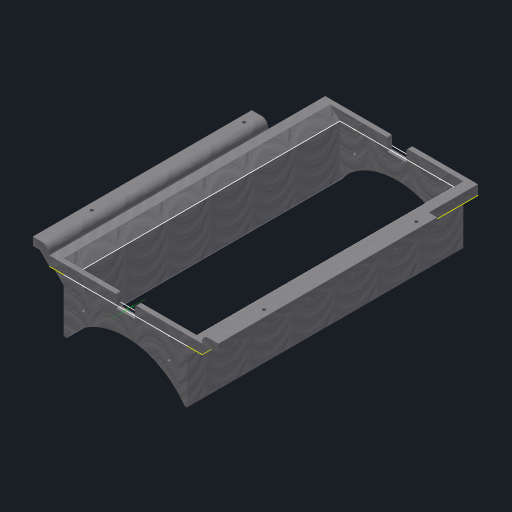
# Autodesk Inventor part: PUERTA_ACOPLE_ENTRADA_v2
Saved by Autodesk Inventor 2024.3 (Build 283343000, 343)
## iProperties
Created: 2024-07-11
Part Number: PUERTA_ACOPLE_ENTRADA_v2
Material: Steel, Mild, Welded
Document SubType Name: Modeling
Designer: Niler
Density: 7.85 g/cm^3
Appearance: Weld - Steel Mild
Author: Niler
Autodesk Inventor part; units mm, degrees
ref_plane "YZ Plane" through (0, 0, 0) normal (1, 0, 0) x (0, 1, 0)
ref_plane "XZ Plane" through (0, 0, 0) normal (0, 1, 0) x (-1, 0, 0)
ref_plane "XY Plane" through (0, 0, 0) normal (0, 0, 1) x (1, 0, 0)
sketch "Sketch1" plane through (0, 0, 0) normal (0, 0, 1) x (1, 0, 0)
  line L0 (-97.5, -4.25) -> (97.5, -4.25)
  line L1 (97.5, -4.25) -> (97.5, 4.25)
  line L2 (97.5, 4.25) -> (-97.5, 4.25)
  line L3 (-97.5, 4.25) -> (-97.5, -4.25)
  line L4 (-97.5, -4.25) -> (97.5, 4.25) construction
  line L5 (97.5, -4.25) -> (-97.5, 4.25) construction
  line L6 (-80.2, 4.25) -> (-80.2, -4.25)
  arc A0 (-80.2, -2.75) -> (-87.2, 4.25) centre (-87.2, -2.75) ccw
  line L7 (0, -4.25) -> (0, 4.25)
  line L8 (97.5, 4.25) -> (97.5, -4.25)
  line L9 (80.2, 4.25) -> (80.2, -4.25)
  arc A1 (87.2, 4.25) -> (80.2, -2.75) centre (87.2, -2.75) ccw
  line L10 (-90.2, -4.25) -> (-80.2, -14.25)
  line L11 (-80.2, -14.25) -> (-0.2084, -14.25)
  line L12 (90.2, -4.25) -> (80.2, -14.25)
  line L13 (80.2, -14.25) -> (0.2084, -14.25)
  line L14 (-65, -14.25) -> (-65, -4.25)
  line L15 (65, -14.25) -> (65, -4.25)
  point P0 (0, 0)
  point P1 (-70, -4.25)
  point P2 (90.2, -4.25)
  point P3 (87.2, 4.25)
  point P4 (80.2, -4.25)
  point P5 (80.2, 4.25)
  dimension "d0" = 195
  dimension "d1" = 8.5
  dimension "d2" = 17.3
  dimension "d3" = 7
  dimension "d4" = 135
  dimension "d5" = 10
  dimension "d8" = 130
  dimension "d11" = 0
  constraints: 32 end point, 11 point on line, 9 symmetric about line, 4 midpoint, 4 perpendicular, 4 point on circle, 2 centre point, 2 horizontal, 2 parallel, 2 tangent, 1 other
  measures "d0" distance of L2.end L1.end
  measures "d1" distance of L1.end L0.end
  measures "d2" distance between parallel lines of L3 L6
  measures "d3" radius of A0
  measures "d4" angle of L11 L10
  measures "d5" distance between parallel lines of L0 L11
  measures "d8" distance of L15.start L14.start
  measures "d11" horizontal distance of L6.end L10.end
extrude "Extrusion1" add sketch "Sketch1" against normal blind 230 contours L3 L2 A0 L6 L0 | L0 L14 L11 L10 | L0 L12 L13 L15 | L9 A1 L2 L1 L0
sketch "Sketch2" plane through (0, 0, -230) normal (0, 0, -1) x (-1, 0, 0)
  line L0 (-80.2, -4.25) -> (-80.2, -2.75) projected
  arc A0 (-80.2, -2.75) -> (-87.2, 4.25) centre (-87.2, -2.75) ccw projected
  line L1 (-87.2, 4.25) -> (-97.5, 4.25) projected
  line L2 (-97.5, 4.25) -> (-97.5, -4.25) projected
  line L3 (-97.5, -4.25) -> (-90.2, -4.25) projected
  line L4 (-90.2, -4.25) -> (-80.2, -14.25) projected
  line L5 (-80.2, -14.25) -> (-65, -14.25) projected
  line L6 (-65, -14.25) -> (-65, -4.25) projected
  line L7 (-65, -4.25) -> (-80.2, -4.25) projected
  line L8 (90.2, -4.25) -> (97.5, -4.25) projected
  line L9 (97.5, -4.25) -> (97.5, 4.25) projected
  line L10 (97.5, 4.25) -> (87.2, 4.25) projected
  arc A1 (87.2, 4.25) -> (80.2, -2.75) centre (87.2, -2.75) ccw projected
  line L11 (80.2, -2.75) -> (80.2, -4.25) projected
  line L12 (80.2, -4.25) -> (65, -4.25) projected
  line L13 (65, -4.25) -> (65, -14.25) projected
  line L14 (65, -14.25) -> (80.2, -14.25) projected
  line L15 (80.2, -14.25) -> (90.2, -4.25) projected
  line L16 (-80.2, -4.25) -> (-80.2, -14.25)
  line L17 (80.2, -4.25) -> (80.2, -14.25)
  point P0 (0, 0)
  constraints: 4 end point, 1 perpendicular, 1 vertical
extrude "Extrusion2" add sketch "Sketch2" along normal blind 60 contours L7 L6 L5 L16 | L14 L13 L12 L17
sketch "Sketch3" plane through (65, -14.25, 0) normal (0, -1, 0) x (1, 0, 0)
  line L0 (0, 0) -> (15.2, 0) projected
  line L1 (0, 0) -> (0, -290) projected
  line L2 (15.2, 0) -> (15.2, -230) projected
  line L3 (-145.2, 0) -> (-130, 0) projected
  line L4 (-145.2, 0) -> (-145.2, -230) projected
  line L5 (-130, 0) -> (-130, -290) projected
  line L6 (0, 0) -> (-130, 0)
  line L7 (-130, 0) -> (-130, -290)
  line L8 (-130, -290) -> (0, -290)
  line L9 (0, -290) -> (0, 0)
  line L10 (-125, -5) -> (-5, -5)
  line L11 (-5, -5) -> (-5, -285)
  line L12 (-5, -285) -> (-125, -285)
  line L13 (-125, -285) -> (-125, -5)
  line L14 (-145.2, -230) -> (-145.2, -290) projected
  line L15 (-130, -290) -> (-145.2, -290) projected
  line L16 (15.2, -290) -> (0, -290) projected
  line L17 (15.2, -230) -> (15.2, -290) projected
  point P0 (-65, 0)
  point P1 (0, -290)
  dimension "d14" = 5
  constraints: 16 end point, 4 parallel, 2 perpendicular, 1 horizontal, 3 other
  measures "d14" distance between parallel lines of L6 L10
extrude "Extrusion3" add sketch "Sketch3" along normal blind 100 contours L1 L8 L5 L6
extrude "Extrusion4" add sketch "Sketch3" against normal up to surface (10 mm away) contours L1 L8 L5 L6
chamfer "Chamfer1" distance 10 angle 45 4 edges at (-60, -4.25, -145) (-65, -14.25, -145) (65, -14.25, -145) (60, -4.25, -145)
sketch "Sketch4" plane through (0, 0, 0) normal (0, 0, 1) x (1, 0, 0)
  line L0 (-97.5, -4.25) -> (-90.2, -4.25) projected
  line L1 (-90.2, -4.25) -> (-80.2, -14.25) projected
  line L2 (-80.2, -14.25) -> (-75, -14.25) projected
  line L3 (-65, -24.25) -> (-75, -14.25) projected
  line L4 (-65, -24.25) -> (-65, -114.25) projected
  line L5 (65, -114.25) -> (-65, -114.25) projected
  line L6 (65, -24.25) -> (65, -114.25) projected
  line L7 (75, -14.25) -> (65, -24.25) projected
  line L8 (75, -14.25) -> (80.2, -14.25) projected
  line L9 (80.2, -14.25) -> (90.2, -4.25) projected
  line L10 (90.2, -4.25) -> (97.5, -4.25) projected
  line L11 (97.5, -4.25) -> (97.5, 4.25) projected
  line L12 (97.5, 4.25) -> (87.2, 4.25) projected
  arc A0 (87.2, 4.25) -> (80.2, -2.75) centre (87.2, -2.75) ccw projected
  line L13 (80.2, -2.75) -> (80.2, -4.25) projected
  line L14 (80.2, -4.25) -> (-80.2, -4.25) projected
  line L15 (-80.2, -4.25) -> (-80.2, -2.75) projected
  arc A1 (-80.2, -2.75) -> (-87.2, 4.25) centre (-87.2, -2.75) ccw projected
  line L16 (-87.2, 4.25) -> (-97.5, 4.25) projected
  line L17 (-97.5, 4.25) -> (-97.5, -4.25) projected
  line L18 (65, -114.25) -> (-65, -114.25) projected
  circle A2 centre (0, -114.25) radius 76
  point P0 (0, 0)
  point P1 (65, -74.8673)
  point P2 (-65, -74.8673)
  dimension "d22" = 152
  constraints: 1 centre point, 1 midpoint
  measures "d22" diameter of A2
extrude "redondo" cut sketch "Sketch4" against normal through all contours A2 L6 L5 L4 picked at (1.9974, -88.9955)
sketch "Sketch5" plane through (-97.5, 4.25, 0) normal (0, 1, 0) x (1, 0, 0)
  line L0 (10.3, 0) -> (0, 0) projected
  line L1 (10.3, 0) -> (10.3, 230) projected
  line L2 (0, 230) -> (10.3, 230) projected
  line L3 (0, 0) -> (0, 230) projected
  line L4 (195, 0) -> (184.7, 0) projected
  line L5 (195, 0) -> (195, 230) projected
  line L6 (184.7, 230) -> (195, 230) projected
  line L7 (184.7, 0) -> (184.7, 230) projected
  circle A0 centre (7, 55) radius 1.65
  line L8 (97.5, 0) -> (97.5, 57.8236)
  circle A1 centre (7, 215) radius 1.65
  circle A2 centre (188, 55) radius 1.65
  circle A3 centre (188, 215) radius 1.65
  dimension "d25" = 3.3
  dimension "d26" = 7
  dimension "d27" = 55
  dimension "d30" = 160
  constraints: 4 centre point, 2 end point, 2 symmetric about line, 2 vertical, 4 other
  measures "d25" diameter of A0
  measures "d26" distance from line of L3 A0.centre
  measures "d27" distance from line of L0 A0.centre
  measures "d30" distance of A0.centre A1.centre
extrude "Extrusion6" cut sketch "Sketch5" against normal through all contours A0 | A1 | A2 | A3
sketch "Sketch6" plane through (-97.5, -4.25, 0) normal (0, -1, 0) x (1, 0, 0)
  arc A0 (7.3, -53.3775) -> (7.3, -56.6225) centre (7, -55) ccw projected
  arc A1 (7.3, -56.6225) -> (7.3, -53.3775) centre (7, -55) ccw projected
  arc A2 (7.3, -213.3775) -> (7.3, -216.6225) centre (7, -215) ccw projected
  arc A3 (7.3, -216.6225) -> (7.3, -213.3775) centre (7, -215) ccw projected
  arc A4 (187.7, -216.6225) -> (187.7, -213.3775) centre (188, -215) ccw projected
  arc A5 (187.7, -213.3775) -> (187.7, -216.6225) centre (188, -215) ccw projected
  arc A6 (187.7, -56.6225) -> (187.7, -53.3775) centre (188, -55) ccw projected
  arc A7 (187.7, -53.3775) -> (187.7, -56.6225) centre (188, -55) ccw projected
  circle A8 centre (188, -55) radius 4
  circle A9 centre (188, -215) radius 4
  circle A10 centre (7, -215) radius 4
  circle A11 centre (7, -55) radius 4
  point P0 (97.5, 0)
  dimension "d37" = 8
  constraints: 4 centre point, 4 coincident, 3 equal radius
  measures "d37" diameter of A8
extrude "Extrusion7" cut sketch "Sketch6" along normal through all
chamfer "Chamfer2" distance 5 angle 45 2 edges at (-65, -74.8673, -145) (65, -74.8673, -145)
sketch "Sketch7" plane through (0, 0, 0) normal (0, 0, 1) x (1, 0, 0)
  arc A0 (62.2698, -70.6785) -> (-62.2698, -70.6785) centre (0, -114.25) ccw projected
  circle A1 centre (0, -114.25) radius 90
  circle A2 centre (-45, -36.3077) radius 1.65
  circle A3 centre (45, -36.3077) radius 1.65
  line L0 (-45, -36.3077) -> (45, -36.3077) construction
  point P0 (0, 0)
  point P1 (0, -36.3077)
  dimension "d43" = 180
  dimension "d44" = 3.3
  dimension "d45" = 3.3
  dimension "d46" = 90
  constraints: 3 centre point, 2 end point, 2 point on circle, 1 coincident, 1 midpoint, 1 vertical alignment
  measures "d43" diameter of A1
  measures "d44" diameter of A2
  measures "d45" diameter of A3
  measures "d46" distance of L0.end L0.start
extrude "Extrusion8" cut sketch "Sketch7" against normal through all contours A3 A1 | A1 A3 | A2 A1 | A1 A2
sketch "Sketch8" plane through (0, 0, 0) normal (0, 0, 1) x (1, 0, 0)
  circle A0 centre (45, -36.3077) radius 1.65 projected
  circle A1 centre (-45, -36.3077) radius 1.65 projected
  line L0 (65, -69.8673) -> (62.2698, -70.6785) projected
  line L1 (65, -24.25) -> (65, -69.8673) projected
  line L2 (75, -14.25) -> (65, -24.25) projected
  line L3 (75, -14.25) -> (80.2, -14.25) projected
  line L4 (80.2, -14.25) -> (90.2, -4.25) projected
  line L5 (90.2, -4.25) -> (97.5, -4.25) projected
  line L6 (97.5, -4.25) -> (97.5, 4.25) projected
  line L7 (97.5, 4.25) -> (87.2, 4.25) projected
  arc A2 (87.2, 4.25) -> (80.2, -2.75) centre (87.2, -2.75) ccw projected
  line L8 (80.2, -2.75) -> (80.2, -4.25) projected
  line L9 (80.2, -4.25) -> (-80.2, -4.25) projected
  line L10 (-80.2, -4.25) -> (-80.2, -2.75) projected
  arc A3 (-80.2, -2.75) -> (-87.2, 4.25) centre (-87.2, -2.75) ccw projected
  line L11 (-87.2, 4.25) -> (-97.5, 4.25) projected
  line L12 (-97.5, 4.25) -> (-97.5, -4.25) projected
  line L13 (-97.5, -4.25) -> (-90.2, -4.25) projected
  line L14 (-90.2, -4.25) -> (-80.2, -14.25) projected
  line L15 (-80.2, -14.25) -> (-75, -14.25) projected
  line L16 (-65, -24.25) -> (-75, -14.25) projected
  line L17 (-65, -24.25) -> (-65, -69.8673) projected
  line L18 (-62.2698, -70.6785) -> (-65, -69.8673) projected
  arc A4 (62.2698, -70.6785) -> (-62.2698, -70.6785) centre (0, -114.25) ccw projected
  line L19 (-10, -4.25) -> (10, -4.25)
  line L20 (10, -4.25) -> (10, -17.25)
  line L21 (10, -17.25) -> (-10, -17.25)
  line L22 (-10, -17.25) -> (-10, -4.25)
  point P0 (0, 0)
  point P1 (0, -17.25)
  point P2 (0, -4.25)
  dimension "d49" = 13
  dimension "d50" = 20
  constraints: 8 end point, 2 midpoint, 2 parallel, 1 horizontal, 1 perpendicular, 1 point on line, 1 vertical alignment
  measures "d49" distance of L19.end L20.end
  measures "d50" distance of L20.end L21.end
extrude "Extrusion9" cut sketch "Sketch8" against normal through all contours L20 L21 L22 L9
fillet "Fillet1" radius 2 4 edges at (-10, -4.25, -2.5) (10, -4.25, -2.5) (10, -4.25, -287.5) (-10, -4.25, -287.5)
sketch "Sketch9" plane through (0, 0, 0) normal (0, 0, 1) x (1, 0, 0)
  arc A0 (12, -4.25) -> (10, -6.25) centre (12, -6.25) ccw projected
  line L0 (10, -6.25) -> (10, -17.25) projected
  line L1 (10, -17.25) -> (-10, -17.25) projected
  line L2 (-10, -17.25) -> (-10, -6.25) projected
  arc A1 (-10, -6.25) -> (-12, -4.25) centre (-12, -6.25) ccw projected
  line L3 (-12, -4.25) -> (-80.2, -4.25) projected
  line L4 (-80.2, -4.25) -> (-80.2, -2.75) projected
  arc A2 (-80.2, -2.75) -> (-87.2, 4.25) centre (-87.2, -2.75) ccw projected
  line L5 (-87.2, 4.25) -> (-97.5, 4.25) projected
  line L6 (-97.5, 4.25) -> (-97.5, -4.25) projected
  line L7 (-97.5, -4.25) -> (-90.2, -4.25) projected
  line L8 (-90.2, -4.25) -> (-80.2, -14.25) projected
  line L9 (-80.2, -14.25) -> (-75, -14.25) projected
  line L10 (-65, -24.25) -> (-75, -14.25) projected
  line L11 (-65, -24.25) -> (-65, -69.8673) projected
  line L12 (-62.2698, -70.6785) -> (-65, -69.8673) projected
  arc A3 (62.2698, -70.6785) -> (-62.2698, -70.6785) centre (0, -114.25) ccw projected
  line L13 (65, -69.8673) -> (62.2698, -70.6785) projected
  line L14 (65, -24.25) -> (65, -69.8673) projected
  line L15 (75, -14.25) -> (65, -24.25) projected
  line L16 (75, -14.25) -> (80.2, -14.25) projected
  line L17 (80.2, -14.25) -> (90.2, -4.25) projected
  line L18 (90.2, -4.25) -> (97.5, -4.25) projected
  line L19 (97.5, -4.25) -> (97.5, 4.25) projected
  line L20 (97.5, 4.25) -> (87.2, 4.25) projected
  arc A4 (87.2, 4.25) -> (80.2, -2.75) centre (87.2, -2.75) ccw projected
  line L21 (80.2, -2.75) -> (80.2, -4.25) projected
  line L22 (80.2, -4.25) -> (12, -4.25) projected
  circle A5 centre (-45, -36.3077) radius 1.65 projected
  circle A6 centre (45, -36.3077) radius 1.65 projected
  circle A7 centre (-45, -14.25) radius 1.65
  circle A8 centre (45, -14.25) radius 1.65
  line L23 (65, -14.25) -> (-65, -14.25) projected
  point P0 (0, 0)
  dimension "d54" = 3.3
  dimension "d55" = 3.3
  constraints: 2 centre point, 2 point on line, 2 vertical alignment
  measures "d54" diameter of A7
  measures "d55" diameter of A8
extrude "Extrusion10" cut sketch "Sketch9" against normal through all contours L23 A7 | A7 L23 | L23 A8 | A8 L23
body "Solid1"
